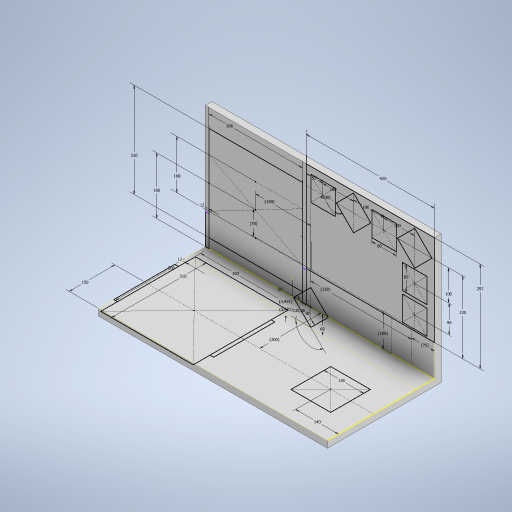
# Autodesk Inventor part: Referenzboard
Saved by Autodesk Inventor 2024 (Build 280153000, 153)
## iProperties
Created: 2024-02-04
Part Number: Referenzboard
Material: Generisch
Document SubType Name: Modeling
Designer: Pavel Povolni
Density: 1 g/cm^3
Appearance: Vorgabe
Author: Pavel Povolni
Autodesk Inventor part; units mm, degrees
ref_plane "YZ Plane" through (0, 0, 0) normal (1, 0, 0) x (0, 1, 0)
ref_plane "XZ Plane" through (0, 0, 0) normal (0, 1, 0) x (-1, 0, 0)
sketch "Skizze1" plane through (0, 0, 0) normal (0, 1, 0) x (-1, 0, 0)
  line L0 (0, 0) -> (-750, 0)
  line L1 (-750, 0) -> (-750, 422)
  line L2 (-750, 422) -> (0, 422)
  line L3 (0, 422) -> (0, 0)
  dimension "d0" = 750
  dimension "d1" = 422
  constraints: 8 end point, 2 parallel, 1 horizontal, 1 perpendicular
  measures "d0" distance of L1.end L2.end
  measures "d1" distance of L0.end L1.end
extrude "Back_Back" add sketch "Skizze1" along normal blind 22
sketch "Skizze2" plane through (0, 0, 0) normal (0, -1, 0) x (1, 0, 0)
  line L0 (750, 422) -> (750, 0) projected
  line L1 (0, 0) -> (750, 0)
  line L2 (750, 0) -> (750, 22)
  line L3 (750, 22) -> (0, 22)
  line L4 (0, 22) -> (0, 0)
  dimension "d4" = 22
  constraints: 8 end point, 2 parallel, 1 horizontal, 1 perpendicular, 1 point on line
  measures "d4" distance between parallel lines of L1 L3
extrude "Back_Down" add sketch "Skizze2" along normal blind 350
sketch "Sketch_Footprint_Magnet&Robot" plane through (0, 0, 22) normal (0, 0, 1) x (1, 0, 0)
  line L0 (0, -350) -> (0, 22) construction
  line L1 (750, -350) -> (0, -350) construction
  line L2 (0, -200) -> (750, -200) construction
  line L3 (12, -45) -> (315, -45)
  line L4 (315, -45) -> (315, -355)
  line L5 (315, -355) -> (12, -355)
  line L6 (12, -355) -> (12, -45)
  line L7 (12, -45) -> (315, -355) construction
  line L8 (315, -45) -> (12, -355) construction
  line L9 (0, -100) -> (12, -100)
  line L10 (12, -100) -> (12, -300)
  line L11 (12, -300) -> (0, -300)
  line L12 (0, -300) -> (0, -100)
  line L13 (315, -100) -> (327, -100)
  line L14 (327, -100) -> (327, -300)
  line L15 (327, -300) -> (315, -300)
  line L16 (315, -300) -> (315, -100)
  line L17 (545, -265) -> (675, -265)
  line L18 (675, -265) -> (675, -135)
  line L19 (675, -135) -> (545, -135)
  line L20 (545, -135) -> (545, -265)
  line L21 (545, -265) -> (675, -135) construction
  line L22 (675, -265) -> (545, -135) construction
  line L23 (750, 0) -> (750, -350) projected
  line L24 (0, 0) -> (750, 0) projected
  point P0 (163.5, -200)
  point P1 (327, -200)
  point P2 (610, -200)
  dimension "d15" = 150
  dimension "d16" = 303
  dimension "d17" = 310
  dimension "d18" = 12
  dimension "d19" = 200
  dimension "d20" = 130
  dimension "d21" = 140
  dimension "d56" = 200
  constraints: 42 end point, 8 parallel, 7 point on line, 5 horizontal, 4 midpoint, 4 perpendicular, 2 collinear, 2 equal length
  measures "d15" distance between parallel lines of L1 L2
  measures "d16" distance of L3.start L3.end
  measures "d17" distance of L5.end L3.start
  measures "d18" distance of L9.start L9.end
  measures "d19" distance of L11.end L9.start
  measures "d20" distance of L18.end L19.end
  measures "d21" distance from line of L23 point (610, -200)
  measures "d56" distance between parallel lines of L2 L24
sketch "Sketch_ReferenceBoard" plane through (0, 0, 0) normal (0, -1, 0) x (1, 0, 0)
  line L0 (750, 422) -> (330, 422)
  line L1 (330, 422) -> (330, 125)
  line L2 (330, 125) -> (750, 125)
  line L3 (750, 125) -> (750, 422)
  line L4 (330, 446) -> (330, 125)
  line L5 (345, 330) -> (345, 130) construction
  line L6 (345, 130) -> (645, 130) construction
  line L7 (345, 208) -> (345, 130)
  line L8 (610, 22) -> (610, 130) construction
  line L9 (675, 22) -> (675, 130) construction
  line L10 (750, 422) -> (750, 22) construction
  line L11 (330, 360) -> (750, 360) construction
  line L12 (685, 422) -> (685, 125) construction
  line L13 (345, 400) -> (425, 400)
  line L14 (425, 400) -> (425, 320)
  line L15 (425, 320) -> (345, 320)
  line L16 (345, 320) -> (345, 400)
  line L17 (345, 400) -> (425, 320) construction
  line L18 (425, 400) -> (345, 320) construction
  line L19 (545, 400) -> (625, 400)
  line L20 (625, 400) -> (625, 320)
  line L21 (625, 320) -> (545, 320)
  line L22 (545, 320) -> (545, 400)
  line L23 (545, 400) -> (625, 320) construction
  line L24 (625, 400) -> (545, 320) construction
  line L25 (645, 220) -> (725, 220)
  line L26 (725, 220) -> (725, 300)
  line L27 (725, 300) -> (645, 300)
  line L28 (645, 300) -> (645, 220)
  line L29 (645, 220) -> (725, 300) construction
  line L30 (725, 220) -> (645, 300) construction
  line L31 (645, 130) -> (725, 130)
  line L32 (725, 130) -> (725, 210)
  line L33 (725, 210) -> (645, 210)
  line L34 (645, 210) -> (645, 130)
  line L35 (645, 130) -> (725, 210) construction
  line L36 (725, 130) -> (645, 210) construction
  line L37 (485, 303.4315) -> (541.5685, 360)
  line L38 (541.5685, 360) -> (485, 416.5685)
  line L39 (485, 416.5685) -> (428.4315, 360)
  line L40 (428.4315, 360) -> (485, 303.4315)
  line L41 (485, 303.4315) -> (485, 416.5685) construction
  line L42 (541.5685, 360) -> (428.4315, 360) construction
  line L43 (685, 303.4315) -> (741.5685, 360)
  line L44 (741.5685, 360) -> (685, 416.5685)
  line L45 (685, 416.5685) -> (628.4315, 360)
  line L46 (628.4315, 360) -> (685, 303.4315)
  line L47 (685, 303.4315) -> (685, 416.5685) construction
  line L48 (741.5685, 360) -> (628.4315, 360) construction
  point P0 (0, 0)
  point P1 (163.5, 22)
  point P2 (685, 360)
  point P3 (585, 360)
  point P4 (485, 360)
  point P5 (385, 360)
  point P6 (685, 260)
  point P7 (685, 170)
  dimension "d7" = 297
  dimension "d8" = 420
  dimension "d24" = 330
  dimension "d25" = 75
  dimension "d26" = 108
  dimension "d28" = 55
  dimension "d29" = 100
  dimension "d30" = 100
  dimension "d31" = 100
  dimension "d32" = 235
  dimension "d33" = 100
  dimension "d34" = 90
  dimension "d35" = 80
  dimension "d36" = 80
  dimension "d37" = 45
  constraints: 96 end point, 16 point on line, 14 parallel, 12 midpoint, 10 perpendicular, 9 equal length, 6 horizontal, 3 collinear, 3 vertical, 1 coincident
  measures "d7" distance of L0.end L1.end
  measures "d8" distance of L1.end L2.end
  measures "d24" distance from line of L9 L7.end
  measures "d25" distance between parallel lines of L10 L9
  measures "d26" distance of L8.start L8.end
  measures "d28" distance from line of L4 point (385, 360)
  measures "d29" distance of point (385, 360) point (485, 360)
  measures "d30" distance of point (485, 360) point (585, 360)
  measures "d31" distance of point (585, 360) point (685, 360)
  measures "d32" distance between parallel lines of L2 L11
  measures "d33" distance of point (685, 260) point (685, 360)
  measures "d34" distance of point (685, 170) point (685, 260)
  measures "d35" distance of L20.end L21.end
  measures "d36" distance of L27.end L25.start
  measures "d37" angle of L14 L40
ref_plane "plane_id6" through (0, -60, 0) normal (0, -1, 0) x (1, 0, 0)
sketch "Sketch_RefrenceBoard_id6" plane through (0, -60, 0) normal (0, -1, 0) x (1, 0, 0)
  line L0 (405, 138.5685) -> (461.5685, 82)
  line L1 (461.5685, 82) -> (405, 25.4315)
  line L2 (405, 25.4315) -> (348.4315, 82)
  line L3 (348.4315, 82) -> (405, 138.5685)
  line L4 (0, 22) -> (750, 22) construction
  line L5 (405, 138.5685) -> (405, 25.4315) construction
  line L6 (348.4315, 82) -> (461.5685, 82) construction
  point P0 (0, 0)
  point P1 (405, 82)
  point P2 (345, 130)
  point P3 (405, 82)
  dimension "d40" = 45
  dimension "d41" = 80
  dimension "d42" = 60
  dimension "d43" = 60
  dimension "d45" = 3.4315
  dimension "d46" = 3.4315
  constraints: 12 end point, 3 perpendicular, 2 midpoint, 2 parallel
  measures "d40" angle of L4 L2
  measures "d41" distance of L1.end L2.end
  measures "d42" horizontal distance of point (405, 82) point (345, 130)
  measures "d43" distance from line of L4 point (405, 82)
  measures "d45" horizontal distance of point (345, 130) L2.end
  measures "d46" distance from line of L4 L1.end
sketch "Sketch_Magnet_Back" plane through (0, 0, 0) normal (0, -1, 0) x (1, 0, 0)
  line L0 (318, 369.7147) -> (318, 209.7147)
  line L1 (12, 209.7147) -> (12, 369.7147)
  line L2 (12, 363) -> (318, 363)
  line L3 (318, 363) -> (318, 53)
  line L4 (318, 53) -> (12, 53)
  line L5 (12, 53) -> (12, 363)
  line L6 (12, 121.0397) -> (0, 121.0397)
  line L7 (0, 121.0397) -> (0, 22)
  line L8 (0, 22) -> (12, 22)
  line L9 (12, 22) -> (12, 121.0397)
  line L10 (318, 121.0397) -> (330, 121.0397)
  line L11 (330, 121.0397) -> (330, 22)
  line L12 (330, 22) -> (318, 22)
  line L13 (318, 22) -> (318, 121.0397)
  line L14 (750, 22) -> (0, 22) construction
  line L15 (0, 22) -> (0, 0) construction
  line L16 (12, 128) -> (318, 128) construction
  line L17 (318, 128) -> (318, 288) construction
  line L18 (318, 288) -> (12, 288) construction
  line L19 (12, 288) -> (12, 128) construction
  line L20 (12, 128) -> (318, 288) construction
  line L21 (318, 128) -> (12, 288) construction
  point P0 (318, 208)
  point P1 (165, 208)
  point P2 (12, 208)
  point P3 (12, 208)
  point P4 (165, 128)
  point P5 (165, 288)
  point P6 (345, 130)
  dimension "d47" = 306
  dimension "d48" = 12
  dimension "d51" = 186
  dimension "d52" = 310
  dimension "d53" = 160
  dimension "d54" = 180
  dimension "d55" = 78
  constraints: 40 end point, 9 parallel, 7 midpoint, 6 collinear, 4 horizontal, 4 perpendicular, 3 point on line, 2 equal length, 2 horizontal alignment
  measures "d47" distance of L2.start L2.end
  measures "d48" distance of L6.start L6.end
  measures "d51" distance from line of L14 point (165, 208)
  measures "d52" distance between parallel lines of L4 L2
  measures "d53" distance of point (165, 128) point (165, 288)
  measures "d54" horizontal distance of point (165, 208) point (345, 130)
  measures "d55" vertical distance of point (345, 130) point (165, 208)
